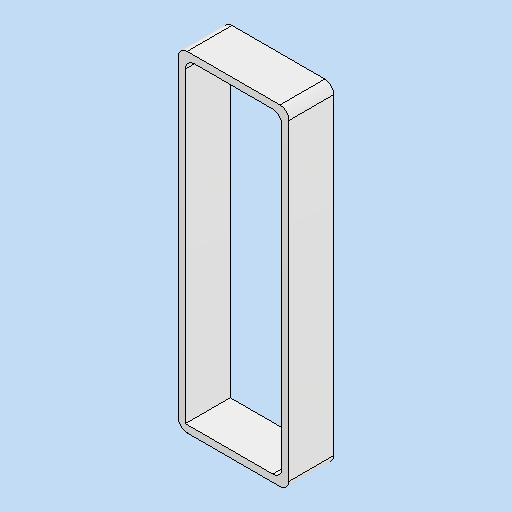
# Autodesk Inventor part: SampleHolderBand
Saved by Autodesk Inventor 2025 (Build 290162000, 162)
## iProperties
Created: 2024-11-07
Part Number: SampleHolderBand
Material: ABS Plastic
Document SubType Name: Modeling
Designer: kuzmin
Density: 1.06 g/cm^3
Appearance: Smooth - White
Author: kuzmin
Autodesk Inventor part; units mm, degrees
ref_plane "YZ Plane" through (0, 0, 0) normal (1, 0, 0) x (0, 1, 0)
ref_plane "XZ Plane" through (0, 0, 0) normal (0, 1, 0) x (-1, 0, 0)
ref_plane "XY Plane" through (0, 0, 0) normal (0, 0, 1) x (1, 0, 0)
sketch "Sketch1" plane through (0, 0, 0) normal (0, 0, 1) x (1, 0, 0)
  line L0 (-10.75, 35.25) -> (10.75, 35.25)
  line L1 (10.75, 35.25) -> (10.75, -35.25)
  line L2 (10.75, -35.25) -> (-10.75, -35.25)
  line L3 (-10.75, -35.25) -> (-10.75, 35.25)
  line L4 (12.35, 36.85) -> (-12.35, 36.85)
  line L5 (-12.35, 36.85) -> (-12.35, -36.85)
  line L6 (-12.35, -36.85) -> (12.35, -36.85)
  line L7 (12.35, -36.85) -> (12.35, 36.85)
  point P0 (0, 0)
  point P1 (10.75, 0)
  point P2 (0, 35.25)
  dimension "d0" = 21.5
  dimension "d1" = 70.5
  dimension "d2" = 1.6
  constraints: 16 end point, 4 parallel, 2 midpoint, 2 perpendicular, 1 horizontal, 1 horizontal alignment, 1 vertical alignment, 3 other
  measures "d0" distance of L0.start L0.end
  measures "d1" distance of L0.end L1.end
  measures "d2" distance between parallel lines of L1 L7
extrude "Extrusion1" add sketch "Sketch1" along normal blind 10
fillet "Fillet1" radius 2 7 edges at (12.35, 36.85, 5) (10.75, 35.25, 5) (-10.75, 35.25, 5) (-12.35, 36.85, 5) (-12.35, -36.85, 5) (12.35, -36.85, 5) (10.75, -35.25, 5)
body "Solid1"
